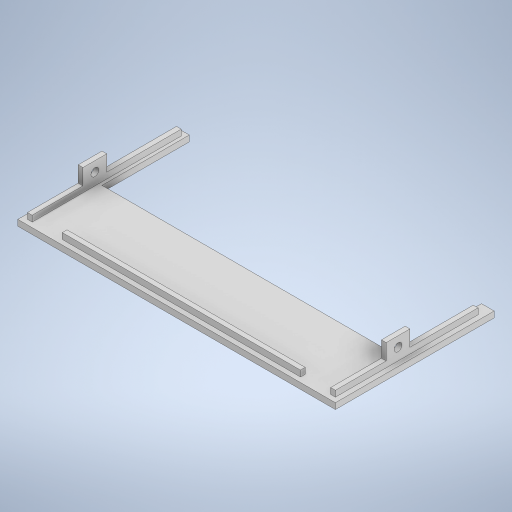
# Autodesk Inventor part: Konsole_Deckel
Saved by Autodesk Inventor 2024 (Build 280153000, 153)
## iProperties
Created: 2024-03-12
Part Number: Konsole_Deckel
Material: Generisch
Document SubType Name: Modeling
Designer: User
Density: 1 g/cm^3
Appearance: Vorgabe
Author: User
Autodesk Inventor part; units mm, degrees
ref_plane "YZ Plane" through (0, 0, 0) normal (1, 0, 0) x (0, 1, 0)
ref_plane "XZ Plane" through (0, 0, 0) normal (0, 1, 0) x (-1, 0, 0)
ref_plane "XY Plane" through (0, 0, 0) normal (0, 0, 1) x (1, 0, 0)
sketch "Skizze1" plane through (0, 0, 0) normal (0, 0, 1) x (1, 0, 0)
  line L0 (-36.1506, 26.4082) -> (43.8494, 26.4082)
  line L1 (43.8494, 26.4082) -> (43.8494, -13.5918)
  line L2 (43.8494, -13.5918) -> (-36.1506, -13.5918)
  line L3 (-36.1506, -13.5918) -> (-36.1506, 26.4082)
  line L4 (-34.9406, 25.1642) -> (-33.7406, 25.1642)
  line L5 (-33.7406, 25.1642) -> (-33.7406, -12.3818)
  line L6 (-33.7406, -12.3818) -> (-34.9406, -12.3818)
  line L7 (-34.9406, -12.3818) -> (-34.9406, 25.1642)
  line L8 (41.4394, 23.5568) -> (42.6394, 23.5568)
  line L9 (42.6394, 23.5568) -> (42.6394, -12.3818)
  line L10 (42.6394, -12.3818) -> (41.4394, -12.3818)
  line L11 (41.4394, -12.3818) -> (41.4394, 23.5568)
  line L12 (-32.9506, 26.4082) -> (40.6494, 26.4082)
  line L13 (40.6494, 26.4082) -> (40.6494, 4.4082)
  line L14 (40.6494, 4.4082) -> (-32.9506, 4.4082)
  line L15 (-32.9506, 4.4082) -> (-32.9506, 26.4082)
  line L16 (-26.1506, -11.1818) -> (33.8494, -11.1818)
  line L17 (33.8494, -11.1818) -> (33.8494, -12.3818)
  line L18 (33.8494, -12.3818) -> (-26.1506, -12.3818)
  line L19 (-26.1506, -12.3818) -> (-26.1506, -11.1818)
  line L20 (42.6394, 0.4082) -> (41.4394, 0.4082)
  line L21 (41.4394, 0.4082) -> (41.4394, 6.4082)
  line L22 (41.4394, 6.4082) -> (42.6394, 6.4082)
  line L23 (42.6394, 6.4082) -> (42.6394, 0.4082)
  line L24 (-33.7406, 0.4082) -> (-34.9406, 0.4082)
  line L25 (-34.9406, 0.4082) -> (-34.9406, 6.4082)
  line L26 (-34.9406, 6.4082) -> (-33.7406, 6.4082)
  line L27 (-33.7406, 6.4082) -> (-33.7406, 0.4082)
  point P0 (0, 0)
  point P1 (-32.9506, 15.4082)
  point P2 (42.0394, -12.3818)
  point P3 (33.8494, -11.7818)
  point P4 (-26.1506, -11.7818)
  point P5 (42.0394, 0.4082)
  point P6 (42.0394, 6.4082)
  point P7 (-34.3406, 0.4082)
  point P8 (-34.3406, 6.4082)
  dimension "d0" = 80
  dimension "d1" = 40
  dimension "d2" = 1.21
  dimension "d3" = 1.21
  dimension "d4" = 35.9386
  dimension "d5" = 1.2
  dimension "d6" = 1.2
  dimension "d7" = 18
  dimension "d8" = 3.2
  dimension "d9" = 3.2
  dimension "d10" = 1.21
  dimension "d11" = 1.21
  dimension "d12" = 1.2
  dimension "d13" = 10
  dimension "d14" = 10
  dimension "d15" = 14
  dimension "d16" = 6
  dimension "d17" = 14
  dimension "d18" = 6
  constraints: 56 end point, 14 parallel, 8 midpoint, 7 horizontal, 7 perpendicular, 6 point on line
  measures "d0" distance of L0.start L0.end
  measures "d1" distance of L2.end L0.start
  measures "d2" distance between parallel lines of L9 L1
  measures "d3" distance between parallel lines of L3 L7
  measures "d4" distance of L8.end L9.end
  measures "d5" distance between parallel lines of L11 L9
  measures "d6" distance between parallel lines of L7 L5
  measures "d7" distance between parallel lines of L2 L14
  measures "d8" distance between parallel lines of L13 L1
  measures "d9" distance from line of L3 point (-32.951, 15.408)
  measures "d10" distance from line of L2 point (42.039, -12.382)
  measures "d11" distance between parallel lines of L2 L18
  measures "d12" distance between parallel lines of L18 L16
  measures "d13" distance from line of L1 point (33.849, -11.782)
  measures "d14" distance from line of L3 point (-26.151, -11.782)
  measures "d15" distance from line of L2 point (42.039, 0.408)
  measures "d16" distance of point (42.039, 0.408) point (42.039, 6.408)
  measures "d17" distance from line of L2 point (-34.341, 0.408)
  measures "d18" distance of point (-34.341, 0.408) point (-34.341, 6.408)
extrude "Extrusion1" add sketch "Skizze1" along normal blind 1.5 contours L0 L15 L14 L13 L1 L2 L3
extrude "Extrusion2" add sketch "Skizze1" along normal blind 3 contours L4 L5 L26 L7 | L24 L5 L6 L7 | L8 L9 L22 L11 | L20 L9 L10 L11 | L16 L17 L18 L19
extrude "Extrusion3" add sketch "Skizze1" along normal blind 7 contours L26 L5 L24 L7 | L22 L9 L20 L11
sketch "Skizze2" plane through (42.6394, -12.3818, 1.5) normal (1, 0, 0) x (0, 0, -1)
  circle A0 centre (-3, 15.79) radius 1
  line L0 (0, -1.21) -> (0, 38.79) projected
  line L1 (1.5, -1.21) -> (0, -1.21) projected
  point P0 (1.5, 12.3818)
  point P1 (0.75, -1.21)
  dimension "d25" = 2
  dimension "d26" = 3
  dimension "d27" = 17
  constraints: 1 centre point, 1 midpoint
  measures "d25" diameter of A0
  measures "d26" distance from line of L0 A0.centre
  measures "d27" vertical distance of point (0.75, -1.21) A0.centre
extrude "Extrusion4" cut sketch "Skizze2" against normal through all
